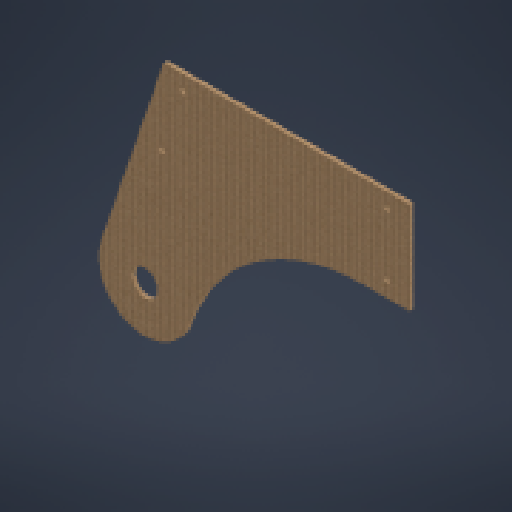
# Autodesk Inventor part: FrameLeg
Saved by Autodesk Inventor 2024.1 (Build 281209000, 209)
## iProperties
Created: 2023-10-16
Part Number: FrameLeg
Material: MDF Medium Density Fiberboard
Document SubType Name: Modeling
Designer: Brandon
Density: 0.8 g/cm^3
Appearance: Cardboard - Corrugated
Author: Brandon
Autodesk Inventor part; units mm, degrees
ref_plane "YZ Plane" through (0, 0, 0) normal (1, 0, 0) x (0, 1, 0)
ref_plane "XZ Plane" through (0, 0, 0) normal (0, 1, 0) x (-1, 0, 0)
ref_plane "XY Plane" through (0, 0, 0) normal (0, 0, 1) x (1, 0, 0)
sketch "Sketch1" plane through (0, 0, 0) normal (0, 0, 1) x (1, 0, 0)
  arc A0 (219.754, -304.8) -> (225.7704, -296.4188) centre (219.754, -298.45) ccw projected
  line L0 (225.7704, -296.4188) -> (30.0819, 283.206) projected
  arc A1 (30.0819, 283.206) -> (-30.0819, 283.206) centre (0, 273.05) ccw projected
  line L1 (-30.0819, 283.206) -> (-225.7704, -296.4188) projected
  arc A2 (-225.7704, -296.4188) -> (-219.754, -304.8) centre (-219.754, -298.45) ccw projected
  line L2 (-219.754, -304.8) -> (219.754, -304.8) projected
  line L3 (-38.1, -17.4222) -> (-38.1, -222.25) projected
  arc A3 (-44.45, -228.6) -> (-38.1, -222.25) centre (-44.45, -222.25) ccw projected
  line L4 (-44.45, -228.6) -> (-113.6024, -228.6) projected
  arc A4 (-119.6188, -220.2188) -> (-113.6024, -228.6) centre (-113.6024, -222.25) ccw projected
  line L5 (-119.6188, -220.2188) -> (-50.4664, -15.391) projected
  arc A5 (-38.1, -17.4222) -> (-50.4664, -15.391) centre (-44.45, -17.4222) ccw projected
  line L6 (113.6024, -228.6) -> (44.45, -228.6) projected
  arc A6 (38.1, -222.25) -> (44.45, -228.6) centre (44.45, -222.25) ccw projected
  line L7 (38.1, -222.25) -> (38.1, -17.4222) projected
  arc A7 (50.4664, -15.391) -> (38.1, -17.4222) centre (44.45, -17.4222) ccw projected
  line L8 (50.4664, -15.391) -> (119.6188, -220.2188) projected
  arc A8 (113.6024, -228.6) -> (119.6188, -220.2188) centre (113.6024, -222.25) ccw projected
  circle A9 centre (-204.2059, -292.1) radius 2 projected
  circle A10 centre (-187.0552, -241.3) radius 2 projected
  circle A11 centre (187.0552, -241.3) radius 2 projected
  circle A12 centre (204.2059, -292.1) radius 2 projected
  circle A13 centre (19.05, -241.3) radius 2 projected
  circle A14 centre (19.05, -292.1) radius 2 projected
  circle A15 centre (-19.05, -292.1) radius 2 projected
  circle A16 centre (-19.05, -241.3) radius 2 projected
  circle A17 centre (8.89, 288.4479) radius 2 projected
  circle A18 centre (-8.89, 288.4479) radius 2 projected
  circle A19 centre (-17.78, 273.05) radius 2 projected
  circle A20 centre (-8.89, 257.6521) radius 2 projected
  circle A21 centre (8.89, 257.6521) radius 2 projected
  circle A22 centre (17.78, 273.05) radius 2 projected
  line L9 (0, -228.6) -> (-202.8739, -228.6)
  line L10 (0, -228.6) -> (0, -304.8)
  line L11 (-119.6188, -220.2188) -> (-208.2019, -482.6)
  line L12 (-225.7704, -296.4188) -> (-288.6275, -482.6)
  line L13 (-288.6275, -482.6) -> (-208.2019, -482.6)
  circle A23 centre (-235.5517, -444.5) radius 38.1
  circle A24 centre (-235.5517, -444.5) radius 10.668
  ellipse E0 centre (0, 273.05) end of major axis (-12.7, 273.05) minor radius 12.2673 projected
  point P0 (0, 0)
  point P1 (-271.6499, -432.3128)
  point P2 (-199.4535, -456.6872)
  point P3 (-148.1744, -304.8)
  dimension "d0" = 21.336
  dimension "d1" = 254
  constraints: 10 end point, 3 collinear, 3 tangent, 2 centre point, 2 horizontal, 2 point on line, 1 coincident, 1 midpoint, 1 other
  measures "d0" diameter of A24
  measures "d1" distance between parallel lines of L13 L9
extrude "Extrusion1" add sketch "Sketch1" along normal blind 3.175 contours L2 L11 L9 L4 L10 | L11 A23 L12 A2 L2 | L2 A2 L1 L9 L11 | A23
fillet "Fillet1" radius 152.4 1 edges at (-148.1744, -304.8, 1.5875)
ref_plane "Work Plane1" through (-235.5517, -444.5, 3.175) normal (0, -0.258819, 0.9659258) x (-1, 0, 0)
sketch "Sketch2" plane through (-235.5517, -444.5, 3.175) normal (0, -0.258819, 0.9659258) x (-1, 0, 0)
  ellipse E0 centre (0, 0) end of major axis (10.668, 0) minor radius 10.3045 projected
  circle A0 centre (0, 0) radius 10.668
  point P0 (-235.5517, -428.5323)
  dimension "d6" = 21.336
  constraints: 1 centre point, 1 coincident
  measures "d6" diameter of A0
sketch "Sketch3" plane through (0, 0, 3.175) normal (0, 0, 1) x (1, 0, 0)
  point P0 (0, 0)
extrude "Extrusion2" cut sketch "Sketch2" along normal through all both and the other way through all
sketch "Sketch4" plane through (0, 0, 3.175) normal (0, 0, 1) x (1, 0, 0)
  ellipse E0 centre (-235.5517, -444.5) end of major axis (-235.5517, -455.5443) minor radius 10.668 (-224.8837, -444.5) -> (-246.2197, -444.5) ccw projected
  ellipse E1 centre (-235.5517, -444.5) end of major axis (-235.5517, -455.5443) minor radius 10.668 (-246.2197, -444.5) -> (-224.8837, -444.5) ccw projected
  line L0 (-202.8739, -228.6) -> (-271.6499, -432.3128) projected
  arc A0 (-271.6499, -432.3128) -> (-199.4535, -456.6872) centre (-235.5517, -444.5) ccw projected
  arc A1 (-38.7755, -304.8) -> (-183.1684, -408.4512) centre (-38.7755, -457.2) ccw projected
  line L1 (-38.7755, -304.8) -> (0, -304.8) projected
  line L2 (0, -304.8) -> (0, -228.6) projected
  line L3 (0, -228.6) -> (-202.8739, -228.6) projected
  circle A2 centre (-19.05, -241.3) radius 2 projected
  circle A3 centre (-19.05, -292.1) radius 2 projected
  circle A4 centre (-204.2059, -292.1) radius 2 projected
  circle A5 centre (-187.0552, -241.3) radius 2 projected
  circle A6 centre (-187.0552, -241.3) radius 2 projected
  circle A7 centre (-204.2059, -292.1) radius 2 projected
  ellipse E2 centre (-235.5517, -443.6493) end of major axis (-235.5517, -454.6936) minor radius 10.668 (-224.8919, -444.082) -> (-246.2115, -444.082) ccw projected
  arc A8 (-246.2115, -444.082) -> (-224.8919, -444.082) centre (-235.5517, -444.5) ccw projected
  circle A9 centre (-19.05, -292.1) radius 2 projected
  circle A10 centre (-19.05, -241.3) radius 2 projected
  line L4 (-202.8739, -228.6) -> (-271.6499, -432.3128) projected
  line L5 (0, -228.6) -> (-202.8739, -228.6) projected
  line L6 (0, -304.8) -> (0, -228.6) projected
  line L7 (-38.7755, -304.8) -> (0, -304.8) projected
  arc A11 (-38.7755, -304.8) -> (-183.1684, -408.4512) centre (-38.7755, -457.2) ccw projected
  arc A12 (-271.6499, -432.3128) -> (-199.4535, -456.6872) centre (-235.5517, -444.5) ccw projected
  line L8 (-199.4535, -456.6872) -> (-183.1684, -408.4512) projected
  line L9 (-199.4535, -456.6872) -> (-183.1684, -408.4512) projected
  point P0 (0, 0)
  constraints: 3 other
extrude "Extrusion3" cut sketch "Sketch4" against normal through all contours A8 E0 | E0 E2
body "Solid1"
